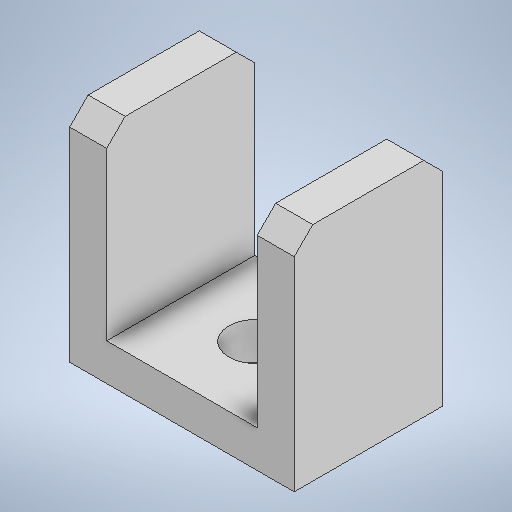
# Autodesk Inventor part: U Bracket
Saved by Autodesk Inventor 2025.1 (Build 291241020, 241B)
## iProperties
Created: 2025-01-11
Part Number: U Bracket
Material: Generic
Document SubType Name: Modeling
Designer: AtuStem
Density: 1 g/cm^3
Appearance: Default
Author: AtuStem
Autodesk Inventor part; units mm, degrees
ref_plane "YZ Plane" through (0, 0, 0) normal (1, 0, 0) x (0, 1, 0)
ref_plane "XZ Plane" through (0, 0, 0) normal (0, 1, 0) x (-1, 0, 0)
ref_plane "XY Plane" through (0, 0, 0) normal (0, 0, 1) x (1, 0, 0)
sketch "Sketch1" plane through (0, 0, 0) normal (0, 0, 1) x (1, 0, 0)
  line L0 (0, 0) -> (19.4056, 0)
  line L1 (0, 0) -> (0, 19.05)
  line L2 (0, 19.05) -> (3.175, 19.05)
  line L3 (3.175, 0) -> (3.175, 3.175)
  line L4 (3.175, 3.175) -> (3.175, 19.05)
  line L5 (3.175, 3.175) -> (9.6266, 3.175)
  line L6 (9.6266, 3.175) -> (9.6266, 0)
  line L7 (19.2532, 0) -> (19.2532, 19.05)
  line L8 (19.2532, 19.05) -> (16.0782, 19.05)
  line L9 (16.0782, 3.175) -> (16.0782, 19.05)
  line L10 (16.0782, 3.175) -> (9.6266, 3.175)
  dimension "d0" = 19.4056
  dimension "d1" = 19.05
  dimension "d2" = 3.175
  dimension "d4" = 3.175
  dimension "d5" = 6.4516
  constraints: 22 end point, 4 symmetric about line, 3 horizontal, 2 point on line, 2 vertical, 1 collinear, 1 perpendicular
  measures "d0" distance of L0.start L0.end
  measures "d1" distance of L0.start L1.end
  measures "d2" distance of L1.end L2.end
  measures "d4" distance of L3.start L3.end
  measures "d5" distance of L3.end L5.end
extrude "Extrusion1" add sketch "Sketch1" along normal blind 12.7
sketch "Sketch2" plane through (3.175, 3.175, 0) normal (0, 1, 0) x (1, 0, 0)
  line L0 (12.9032, 0) -> (0, 0) projected
  line L1 (0, 0) -> (0, -12.7) projected
  line L2 (12.9032, -12.7) -> (0, -12.7) projected
  line L3 (12.9032, 0) -> (12.9032, -12.7) projected
  line L4 (0, 0) -> (6.4516, 0)
  line L5 (12.9032, 0) -> (0, 0) projected
  line L6 (6.4516, 0) -> (6.4516, -6.35)
  circle A0 centre (6.4516, -6.35) radius 2.3241
  point P0 (-3.175, 0)
  dimension "d8" = 6.4516
  dimension "d9" = 6.35
  dimension "d10" = 4.6482
  constraints: 4 end point, 1 centre point, 1 coincident, 1 midpoint, 1 vertical
  measures "d8" distance of L0.end L4.end
  measures "d9" distance of L4.end L6.end
  measures "d10" diameter of A0
extrude "Extrusion2" cut sketch "Sketch2" against normal blind 12.7 contours A0
chamfer "Chamfer1" distance 1.5875 angle 45 4 edges at (1.5875, 19.05, 0) (1.5875, 19.05, 12.7) (17.6657, 19.05, 12.7) (17.6657, 19.05, 0)
body "Solid1"
